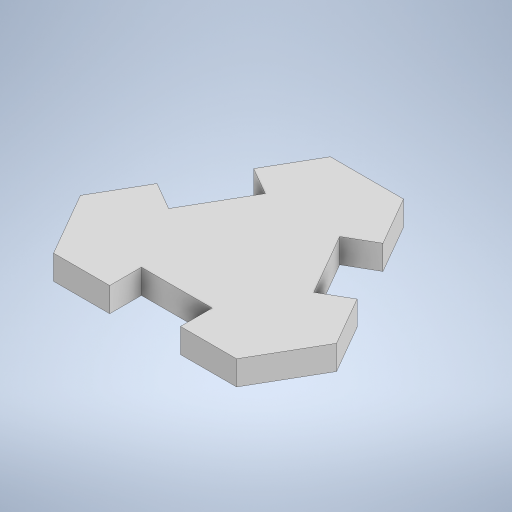
# Autodesk Inventor part: base_flame
Saved by Autodesk Inventor 2024.1 (Build 281209000, 209)
## iProperties
Created: 2025-03-10
Part Number: base_flame
Material: 一般
Document SubType Name: Modeling
Designer: hibik
Density: 1 g/cm^3
Appearance: 既定
Author: hibik
Autodesk Inventor part; units mm, degrees
ref_plane "YZ Plane" through (0, 0, 0) normal (1, 0, 0) x (0, 1, 0)
ref_plane "XZ Plane" through (0, 0, 0) normal (0, 1, 0) x (-1, 0, 0)
ref_plane "XY Plane" through (0, 0, 0) normal (0, 0, 1) x (1, 0, 0)
sketch "スケッチ1" plane through (0, 0, 0) normal (0, 1, 0) x (-1, 0, 0)
  line L0 (135, 77.9423) -> (-135, 77.9423)
  line L1 (-135, 77.9423) -> (0, -155.8846)
  line L2 (0, -155.8846) -> (135, 77.9423)
  line L3 (135, 77.9423) -> (-67.5, -38.9711) construction
  line L4 (75, 77.9423) -> (105, 25.9808)
  line L5 (-105, 25.9808) -> (-75, 77.9423)
  line L6 (30, -103.923) -> (-30, -103.923)
  line L7 (77.8868, 82.9423) -> (0, 82.9423)
  line L8 (77.8868, 82.9423) -> (94.3301, 54.4615)
  line L9 (0, 0) -> (0, 82.9423) construction
  line L10 (-77.8868, 82.9423) -> (0, 82.9423)
  line L11 (-77.8868, 82.9423) -> (-94.3301, 54.4615)
  line L12 (-110.7735, 25.9808) -> (-94.3301, 54.4615)
  line L13 (-110.7735, 25.9808) -> (-71.8301, -41.4711)
  line L14 (-32.8868, -108.923) -> (-71.8301, -41.4711)
  line L15 (-32.8868, -108.923) -> (0, -108.923)
  line L16 (32.8868, -108.923) -> (0, -108.923)
  line L17 (32.8868, -108.923) -> (71.8301, -41.4711)
  line L18 (110.7735, 25.9808) -> (71.8301, -41.4711)
  line L19 (110.7735, 25.9808) -> (94.3301, 54.4615)
  line L20 (30, -108.923) -> (30, -103.923)
  line L21 (-30, -108.923) -> (-30, -103.923)
  line L22 (-30, -103.923) -> (30, -103.923)
  dimension "d0" = 270
  dimension "d1" = 60
  dimension "d4" = 360
  dimension "d6" = 5
  dimension "d7" = 5
  dimension "d10" = 360
  constraints: 46 end point, 9 point on line, 3 parallel, 3 perpendicular, 2 equal length, 2 symmetric about line, 2 vertical alignment, 1 horizontal, 1 midpoint, 1 vertical, 38 other
  measures "d0" distance of L0.start L0.end
  measures "d1" distance of L0.start L4.start
  measures "d6" distance between parallel lines of L7 L0
  measures "d7" distance between parallel lines of L4 L8
extrude "押し出し2" add sketch "スケッチ1" along normal blind 20 contours L4 L2 L6 L1 L5 L0
sketch "スケッチ2" plane through (0, 20, 0) normal (0, 1, 0) x (1, 0, 0)
  line L0 (-75, -77.9423) -> (75, -77.9423) projected
  line L1 (-29, -77.9423) -> (29, -77.9423)
  line L2 (29, -77.9423) -> (29, -51.9423)
  line L3 (29, -51.9423) -> (-29, -51.9423)
  line L4 (-29, -51.9423) -> (-29, -77.9423)
  point P0 (0, 0)
  point P1 (0, -51.9423)
  point P2 (0, -77.9423)
  dimension "d16" = 26
  dimension "d17" = 58
  constraints: 8 end point, 2 midpoint, 2 parallel, 1 horizontal, 1 perpendicular, 1 point on line, 1 vertical alignment
  measures "d16" distance of L3.end L1.start
  measures "d17" distance of L2.end L3.end
extrude "押し出し3" cut sketch "スケッチ2" against normal blind 20
pattern_circular "円形状パターン1" count 3 over 360 about axis through (0, -10, 0) along (0, 1, 0) of "押し出し3"
